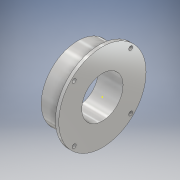
# Autodesk Inventor part: Sleeve Endcap
Saved by Autodesk Inventor 2017.3 (Build 213256000, 256)
## iProperties
Created: 2017-02-08
Part Number: Sleeve Endcap
Material: Generic
Document SubType Name: Modeling
Designer: Mac
Density: 1 g/cm^3
Appearance: Aluminum - Dark
Author: Mac
Autodesk Inventor part; units mm, degrees
ref_plane "YZ Plane" through (0, 0, 0) normal (1, 0, 0) x (0, 1, 0)
ref_plane "XZ Plane" through (0, 0, 0) normal (0, 1, 0) x (-1, 0, 0)
ref_plane "XY Plane" through (0, 0, 0) normal (0, 0, 1) x (1, 0, 0)
sketch "Sketch1" plane through (0, 0, 0) normal (1, 0, 0) x (0, 1, 0)
  circle A0 centre (0, 0) radius 13.2
  dimension "d0" = 26.4
  constraints: 1 centre point, 1 coincident
  measures "d0" diameter of A0
extrude "Extrusion1" add sketch "Sketch1" along normal blind 1
sketch "Sketch2" plane through (0, 0, 0) normal (-1, 0, 0) x (0, 0, 1)
  circle A0 centre (0, 0) radius 11
  dimension "d3" = 22
  constraints: 1 centre point, 1 coincident
  measures "d3" diameter of A0
extrude "Extrusion2" add sketch "Sketch2" along normal blind 6.5
sketch "Sketch3" plane through (1, 0, 0) normal (1, 0, 0) x (0, 0, -1)
  point P0 (0, 0)
  point P1 (8.556, 8.556)
  point P2 (8.556, -8.556)
  point P3 (-8.556, 8.556)
  point P4 (-8.556, -8.556)
hole "Hole1" at (1, 8.556, -8.556) at (1, -8.556, -8.556) at (1, 8.556, 8.556) at (1, -8.556, 8.556) direction (-1, 0, 0) diameter 1.221 depth 5.3 tip angle 118
sketch "Sketch4" plane through (1, 0, 0) normal (1, 0, 0) x (0, 0, -1)
  point P0 (0, 0)
sketch "Sketch5" plane through (-6.5, 0, 0) normal (-1, 0, 0) x (0, 0, 1)
  circle A0 centre (3.905, 6.764) radius 0.835
  circle A1 centre (-3.905, 6.764) radius 0.835
  circle A2 centre (-7.81, 0) radius 0.835
  circle A3 centre (7.81, 0) radius 0.835
  circle A4 centre (3.905, -6.764) radius 0.835
  circle A5 centre (-3.905, -6.764) radius 0.835
  point P0 (0, 0)
  dimension "d13" = 1.67
  dimension "d14" = 1.67
  dimension "d15" = 1.67
  dimension "d16" = 1.67
  dimension "d17" = 1.67
  dimension "d18" = 1.67
  constraints: 6 centre point
  measures "d13" diameter of A0
  measures "d14" diameter of A1
  measures "d15" diameter of A2
  measures "d16" diameter of A3
  measures "d17" diameter of A4
  measures "d18" diameter of A5
extrude "Extrusion3" cut sketch "Sketch5" against normal blind 1
sketch "Sketch6" plane through (-6.5, 0, 0) normal (-1, 0, 0) x (0, 0, 1)
  circle A0 centre (0, 0) radius 6.25
  dimension "d21" = 12.5
  constraints: 1 centre point, 1 coincident
  measures "d21" diameter of A0
extrude "Extrusion4" cut sketch "Sketch6" against normal blind 10
body "Solid1"
